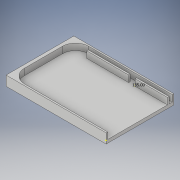
# Autodesk Inventor part: Playfield
Saved by Autodesk Inventor 2018 (Build 220112000, 112)
## iProperties
Created: 2018-10-08
Part Number: Playfield
Material: Generic
Document SubType Name: Modeling
Designer: zdaly3183
Density: 1 g/cm^3
Appearance: Default
Author: zdaly3183
Autodesk Inventor part; units mm, degrees
ref_plane "YZ Plane" through (0, 0, 0) normal (1, 0, 0) x (0, 1, 0)
ref_plane "XZ Plane" through (0, 0, 0) normal (0, 1, 0) x (-1, 0, 0)
ref_plane "XY Plane" through (0, 0, 0) normal (0, 0, 1) x (1, 0, 0)
sketch "Sketch1" plane through (0, 0, 0) normal (0, 1, 0) x (-1, 0, 0)
  line L0 (0, 0) -> (787.4, 0)
  line L1 (787.4, 0) -> (787.4, -533.4)
  line L2 (787.4, -533.4) -> (0, -533.4)
  line L3 (0, -533.4) -> (0, 0)
  dimension "d0" = 787.4
  dimension "d1" = 533.4
  constraints: 8 end point, 2 parallel, 1 horizontal, 1 perpendicular
  measures "d0" distance of L1.end L2.end
  measures "d1" distance of L0.end L1.end
extrude "Extrusion1" add sketch "Sketch1" along normal blind 25.4
sketch "Sketch2" plane through (0, 25.4, 0) normal (0, 1, 0) x (1, 0, 0)
  line L0 (-787.4, 0) -> (0, 0) projected
  line L1 (-787.4, 533.4) -> (-787.4, 0) projected
  line L2 (0, 0) -> (-787.4, 0)
  line L3 (-787.4, 0) -> (-787.4, 12.7)
  line L4 (-787.4, 12.7) -> (0, 12.7)
  line L5 (0, 12.7) -> (0, 0)
  line L6 (0, 533.4) -> (-787.4, 533.4) projected
  line L7 (0, 0) -> (0, 533.4) projected
  line L8 (-787.4, 533.4) -> (0, 533.4)
  line L9 (0, 533.4) -> (0, 520.7)
  line L10 (0, 520.7) -> (-787.4, 520.7)
  line L11 (-787.4, 520.7) -> (-787.4, 533.4)
  line L12 (-787.4, 533.4) -> (-762, 533.4)
  line L13 (-762, 533.4) -> (-762, 0)
  line L14 (-762, 0) -> (-787.4, 0)
  line L15 (-787.4, 0) -> (-787.4, 533.4)
  dimension "d4" = 12.7
  dimension "d5" = 12.7
  dimension "d6" = 25.4
  constraints: 24 end point, 6 parallel, 3 horizontal, 3 perpendicular, 3 point on line
  measures "d4" distance of L2.end L3.end
  measures "d5" distance of L8.end L9.end
  measures "d6" distance of L13.end L14.end
extrude "Extrusion2" add sketch "Sketch2" along normal blind 50.8 contours L1 L4 L13 L0 | L13 L4 L5 L0 | L1 L10 L13 L4 | L1 L6 L13 L10 | L13 L6 L7 L10
sketch "Sketch3" plane through (0, 25.4, 0) normal (0, 1, 0) x (1, 0, 0)
  line L0 (0, 533.4) -> (-787.4, 533.4) construction
  line L1 (0, 533.4) -> (0, 520.7) construction
  line L2 (0, 533.4) -> (0, 0) construction
  line L3 (0, 12.7) -> (0, 520.7) construction
  line L4 (0, 520.7) -> (0, 495.3) construction
  line L5 (-762, 520.7) -> (-762, 12.7) construction
  line L6 (-762, 520.7) -> (-762, 495.3) construction
  line L7 (0, 520.7) -> (-762, 520.7) construction
  line L8 (-762, 520.7) -> (-762, 419.1) construction
  line L9 (-762, 520.7) -> (-660.4, 520.7) construction
  arc A0 (-660.4, 520.7) -> (-762, 419.1) centre (-660.4, 419.1) ccw construction
  line L10 (0, 495.3) -> (-660.4, 495.3)
  line L11 (-660.4, 495.3) -> (-660.4, 482.6)
  line L12 (-660.4, 482.6) -> (0, 482.6)
  line L13 (0, 482.6) -> (0, 495.3)
  arc A1 (-660.4, 520.7) -> (-762, 419.1) centre (-660.4, 419.1) ccw
  line L14 (-762, 419.1) -> (-762, 520.7)
  line L15 (-762, 520.7) -> (-660.4, 520.7)
  dimension "d9" = 12.7
  dimension "d10" = 25.4
  dimension "d11" = 25.4
  dimension "d12" = 101.6
  dimension "d13" = 101.6
  dimension "d14" = 12.7
  constraints: 22 end point, 5 point on line, 4 point on circle, 2 centre point, 2 parallel, 2 tangent, 1 coincident, 1 collinear, 1 horizontal, 1 perpendicular
  measures "d9" distance of L0.start L1.end
  measures "d10" distance of L1.end L4.end
  measures "d11" distance of L5.start L6.end
  measures "d12" distance of L5.start L8.end
  measures "d13" distance of L5.start L9.end
  measures "d14" distance of L11.end L10.end
extrude "Extrusion3" add sketch "Sketch3" along normal blind 50.8
sketch "Sketch4" plane through (0, 25.4, 0) normal (0, 1, 0) x (1, 0, 0)
  line L0 (0, 12.7) -> (-762, 12.7) construction
  line L1 (-762, 12.7) -> (-654.2369, 120.4631) construction
  line L2 (-762, 12.7) -> (-609.6, 12.7) construction
  line L3 (-762, 419.1) -> (-762, 12.7) projected
  arc A0 (-762, 120.4631) -> (-654.2369, 12.7) centre (-654.2369, 120.4631) ccw
  line L4 (-654.2369, 12.7) -> (-762, 12.7)
  line L5 (-762, 120.4631) -> (-762, 12.7)
  point P0 (0, 0)
  dimension "d18" = 152.4
  dimension "d19" = 45
  constraints: 8 end point, 2 horizontal, 2 point on circle, 2 point on line, 1 centre point, 1 coincident, 1 equal length, 1 perpendicular, 1 tangent
  measures "d18" distance of L0.end L1.end
  measures "d19" angle of L2 L1
extrude "Extrusion4" add sketch "Sketch4" along normal blind 50.8
sketch "Sketch6" plane through (0, 76.2, 0) normal (0, 1, 0) x (1, 0, 0)
  line L0 (-660.4, 482.6) -> (0, 482.6) projected
  line L1 (-254.5688, 482.6) -> (-254.5688, 495.3)
  line L2 (0, 495.3) -> (-660.4, 495.3) projected
  line L3 (-254.5688, 482.6) -> (-305.3688, 482.6)
  line L4 (-305.3688, 482.6) -> (-305.3688, 495.3)
  line L5 (-305.3688, 495.3) -> (-254.5688, 495.3)
  point P0 (0, 0)
  dimension "d22" = 50.8
  constraints: 8 end point, 4 point on line, 1 collinear, 1 perpendicular, 1 vertical
  measures "d22" distance of L1.start L3.end
extrude "Extrusion5" cut sketch "Sketch6" against normal blind 50.8
sketch "Sketch8" plane through (0, 76.2, 0) normal (0, 1, 0) x (1, 0, 0)
  line L0 (-305.3688, 482.6) -> (-660.4, 482.6) projected
  line L1 (-660.4, 482.6) -> (-635, 482.6)
  line L2 (-635, 482.6) -> (-635, 495.3)
  line L3 (-305.3688, 495.3) -> (-660.4, 495.3) projected
  line L4 (-660.4, 495.3) -> (-635, 495.3)
  line L5 (-660.4, 482.6) -> (-660.4, 495.3) projected
  line L6 (-660.4, 482.6) -> (-660.4, 495.3)
  point P0 (0, 0)
  dimension "d26" = 25.4
  constraints: 8 end point, 2 collinear, 2 point on line, 1 perpendicular
  measures "d26" distance of L0.end L1.end
extrude "Extrusion6" cut sketch "Sketch8" against normal blind 50.8
sketch "Sketch7" plane through (0, 25.4, 0) normal (0, 1, 0) x (1, 0, 0)
  line L0 (-254.5688, 495.3) -> (-279.9688, 520.7) construction
  line L1 (0, 520.7) -> (-660.4, 520.7) construction
  line L2 (-254.5688, 495.3) -> (-218.6478, 495.3) construction
  point P0 (0, 0)
  dimension "d25" = 135
  constraints: 4 end point, 1 equal length, 1 horizontal, 1 point on line
  measures "d25" angle of L2 L0
sketch "Sketch9" plane through (0, 25.4, 0) normal (0, 1, 0) x (1, 0, 0)
  line L0 (0, 520.7) -> (-660.4, 520.7) construction
  line L1 (-635, 495.3) -> (-305.3688, 495.3) construction
  line L2 (-660.4, 520.7) -> (-635, 495.3) construction
  point P0 (0, 0)
  constraints: 2 end point
body "Solid1"
